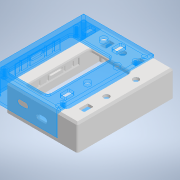
# Autodesk Inventor part: Frontpanel
Saved by Autodesk Inventor 2022 (Build 260153000, 153)
## iProperties
Created: 2020-11-05
Part Number: Frontpanel
Material: Generic
Document SubType Name: Modeling
Designer: simen
Density: 1 g/cm^3
Appearance: Default
Mass: 47.3769 g
Surface Area: 341.342 cm^2
Volume: 47.3769 cm^3
Author: simen
Autodesk Inventor part; units mm, degrees
ref_plane "YZ Plane" through (0, 0, 0) normal (1, 0, 0) x (0, 1, 0)
ref_plane "XZ Plane" through (0, 0, 0) normal (0, 1, 0) x (-1, 0, 0)
ref_plane "XY Plane" through (0, 0, 0) normal (0, 0, 1) x (1, 0, 0)
sketch "Sketch1" plane through (0, 0, 0) normal (0, 1, 0) x (-1, 0, 0)
  line L0 (-18.2777, 28.6513) -> (-98.2777, 28.6513)
  line L1 (-98.2777, 28.6513) -> (-98.2777, -79.3487)
  line L2 (-98.2777, -79.3487) -> (-18.2777, -79.3487)
  line L3 (-18.2777, -79.3487) -> (-18.2777, 28.6513)
  point P0 (0, 0)
  dimension "d0" = 80
  dimension "d42" = 108
  constraints: 8 end point, 2 parallel, 1 horizontal, 1 perpendicular
  measures "d0" distance of L2.end L1.end
  measures "d42" distance of L0.end L1.end
extrude "Extrusion1" add sketch "Sketch1" along normal blind 3
sketch "Sketch2" plane through (0, 3, 0) normal (0, 1, 0) x (1, 0, 0)
  line L0 (23.2777, -23.6513) -> (72.1777, -23.6513)
  line L1 (72.1777, -23.6513) -> (72.1777, 49.7887)
  line L2 (72.1777, 49.7887) -> (23.2777, 49.7887)
  line L3 (23.2777, 49.7887) -> (23.2777, -23.6513)
  line L4 (18.2777, 79.3487) -> (18.2777, -28.6513) projected
  line L5 (18.2777, -28.6513) -> (98.2777, -28.6513) projected
  line L6 (98.2777, 79.3487) -> (18.2777, 79.3487) projected
  point P0 (0, 0)
  dimension "d5" = 5
  dimension "d6" = 5
  dimension "d8" = 48.9
  dimension "d9" = 73.44
  constraints: 8 end point, 2 parallel, 1 horizontal, 1 perpendicular
  measures "d5" distance between parallel lines of L4 L3
  measures "d6" distance between parallel lines of L5 L0
  measures "d8" distance of L0.start L0.end
  measures "d9" distance between parallel lines of L2 L0
extrude "Extrusion2" [suppressed]
sketch "Sketch5" plane through (0, 0, 0) normal (0, -1, 0) x (1, 0, 0)
  line L0 (98.2777, 28.6513) -> (98.2777, -79.3487) projected
  line L1 (18.2777, 28.6513) -> (98.2777, 28.6513) projected
  line L2 (18.2777, -79.3487) -> (18.2777, 28.6513) projected
  line L3 (98.2777, -79.3487) -> (18.2777, -79.3487) projected
  line L4 (95.2777, 25.6513) -> (95.2777, -76.3487)
  line L5 (95.2777, -76.3487) -> (21.2777, -76.3487)
  line L6 (21.2777, -76.3487) -> (21.2777, 25.6513)
  line L7 (21.2777, 25.6513) -> (95.2777, 25.6513)
  point P0 (0, 0)
  dimension "d26" = 3
  constraints: 8 end point, 3 other
  measures "d26" distance between parallel lines of L1 L7
extrude "Extrusion7" add sketch "Sketch5" along normal blind 26
chamfer "Chamfer2" [suppressed]
fillet "Fillet2" radius 2 4 edges at (18.2777, -11.5, -79.3487) (98.2777, -11.5, -79.3487) (98.2777, -11.5, 28.6513) (18.2777, -11.5, 28.6513)
sketch "Sketch8" plane through (18.2777, -26, -77.3487) normal (-1, 0, 0) x (0, 0, 1)
  line L0 (57, 14.5) -> (47, 14.5) construction
  line L1 (57, 17) -> (47, 17)
  line L2 (47, 12) -> (57, 12)
  arc A0 (57, 12) -> (57, 17) centre (57, 14.5) ccw
  arc A1 (47, 17) -> (47, 12) centre (47, 14.5) ccw
  line L3 (0, 0) -> (0, 29) projected
  line L4 (104, 0) -> (0, 0) projected
  line L5 (104, 29) -> (104, 0) projected
  line L6 (104, 0) -> (0, 0) construction
  line L7 (48.7646, 0) -> (45.2354, 29) construction
  line L8 (0, 29) -> (104, 29) projected
  line L9 (0, 29) -> (104, 29) construction
  line L10 (104, 0) -> (0, 29) construction
  line L11 (0, 0) -> (0, 29) construction
  line L12 (0, 0) -> (104, 29) construction
  point P0 (52, 14.5)
  point P1 (52, 14.5)
  dimension "d51" = 10
  dimension "d52" = 5
  constraints: 14 end point, 4 point on circle, 4 tangent, 3 midpoint, 2 centre point, 1 coincident, 1 horizontal, 1 parallel, 1 point on line
  measures "d51" distance of L0.end L0.start
  measures "d52" diameter of A1
extrude "Extrusion9" cut sketch "Sketch8" against normal blind 10 contours A0 L2 A1 L1
sketch "Sketch9" plane through (0, 3, 0) normal (0, 1, 0) x (1, 0, 0)
  line L0 (35.2777, -20.6513) -> (75.2777, -20.6513)
  line L1 (78.2777, -17.6513) -> (78.2777, 48.3487)
  line L2 (75.2777, 51.3487) -> (35.2777, 51.3487)
  line L3 (32.2777, 48.3487) -> (32.2777, -17.6513)
  line L4 (18.2777, 69.3487) -> (18.2777, -25.6513) projected
  arc A0 (32.2777, -17.6513) -> (35.2777, -20.6513) centre (35.2777, -17.6513) ccw
  arc A1 (75.2777, -20.6513) -> (78.2777, -17.6513) centre (75.2777, -17.6513) ccw
  arc A2 (78.2777, 48.3487) -> (75.2777, 51.3487) centre (75.2777, 48.3487) ccw
  arc A3 (35.2777, 51.3487) -> (32.2777, 48.3487) centre (35.2777, 48.3487) ccw
  line L5 (98.2777, -26.6513) -> (98.2777, 77.3487) projected
  line L6 (20.2777, -28.6513) -> (96.2777, -28.6513) projected
  point P0 (0, 0)
  point P1 (78.2777, 51.3487)
  point P2 (78.2777, -20.6513)
  point P3 (32.2777, 51.3487)
  dimension "d56" = 46
  dimension "d57" = 72
  dimension "d59" = 14
  dimension "d60" = 3
  dimension "d116" = 20
  dimension "d144" = 8
  constraints: 8 end point, 8 point on circle, 8 tangent, 6 point on line, 4 centre point, 3 equal radius, 2 parallel, 1 horizontal, 1 perpendicular
  measures "d56" distance of point (32.278, 51.349) point (78.278, 51.349)
  measures "d57" distance of point (78.278, 51.349) point (78.278, -20.651)
  measures "d59" distance between parallel lines of L4 L3
  measures "d60" radius of A0
  measures "d116" distance between parallel lines of L5 L1
  measures "d144" distance between parallel lines of L6 L0
extrude "Extrusion10" cut sketch "Sketch9" against normal blind 10
chamfer "Chamfer4" distance 1 angle 45 8 edges at (33.1563, 3, 19.7726) (32.2777, 3, -15.3487) (33.1563, 3, -50.4701) (55.2777, 3, -51.3487) (77.399, 3, -50.4701) (78.2777, 3, -15.3487) (77.399, 3, 19.7726) (55.2777, 3, 20.6513)
chamfer "Chamfer5" distance 2 angle 45 8 edges at (98.2777, 3, -25.3487) (97.6919, 3, -78.763) (58.2777, 3, -79.3487) (18.8635, 3, -78.763) (18.2777, 3, -25.3487) (18.8635, 3, 28.0655) (58.2777, 3, 28.6513) (97.6919, 3, 28.0655)
fillet "Fillet3" radius 2 8 edges at (95.2777, -13, 25.6513) (95.2777, 0, -25.3487) (58.2777, 0, 25.6513) (95.2777, -13, -76.3487) (58.2777, 0, -76.3487) (21.2777, -13, -76.3487) (21.2777, 0, -25.3487) (21.2777, -13, 25.6513)
sketch "Sketch10" plane through (0, 3, 0) normal (0, 1, 0) x (1, 0, 0)
  arc A0 (31.2777, -17.6513) -> (35.2777, -21.6513) centre (35.2777, -17.6513) ccw projected
  line L0 (31.2777, 48.3487) -> (31.2777, -17.6513) projected
  arc A1 (35.2777, 52.3487) -> (31.2777, 48.3487) centre (35.2777, 48.3487) ccw projected
  line L1 (75.2777, 52.3487) -> (35.2777, 52.3487) projected
  arc A2 (79.2777, 48.3487) -> (75.2777, 52.3487) centre (75.2777, 48.3487) ccw projected
  line L2 (79.2777, -17.6513) -> (79.2777, 48.3487) projected
  arc A3 (75.2777, -21.6513) -> (79.2777, -17.6513) centre (75.2777, -17.6513) ccw projected
  line L3 (35.2777, -21.6513) -> (75.2777, -21.6513) projected
  line L4 (96.2777, -26.6513) -> (20.2777, -26.6513) projected
  line L5 (96.2777, 77.3487) -> (96.2777, -26.6513) projected
  line L6 (20.2777, 77.3487) -> (96.2777, 77.3487) projected
  line L7 (20.2777, -26.6513) -> (20.2777, 77.3487) projected
  arc A4 (75.2777, -21.6513) -> (79.2777, -17.6513) centre (75.2777, -17.6513) ccw projected
  line L8 (79.2777, -17.6513) -> (96.2777, -17.6513) construction
  line L9 (87.7777, -17.6513) -> (87.7777, -7.6513) construction
  circle A5 centre (87.7777, -7.6513) radius 2
  line L10 (87.7777, -7.6513) -> (87.7777, 17.3487) construction
  circle A6 centre (87.7777, 17.3487) radius 2
  point P0 (0, 0)
  dimension "d70" = 10
  dimension "d71" = 4
  dimension "d72" = 25
  dimension "d73" = 4
  constraints: 6 end point, 2 centre point, 2 coincident, 2 perpendicular, 1 collinear, 1 midpoint, 1 point on line
  measures "d70" distance of L9.start L9.end
  measures "d71" diameter of A5
  measures "d72" distance of L10.start L10.end
  measures "d73" diameter of A6
extrude "Extrusion11" [suppressed]
sketch "Sketch11" plane through (0, 0, 0) normal (0, -1, 0) x (1, 0, 0)
  circle A0 centre (92.2777, 22.6513) radius 2.5
  line L0 (95.2777, 23.6513) -> (95.2777, -74.3487) projected
  line L1 (23.2777, 25.6513) -> (93.2777, 25.6513) projected
  circle A1 centre (92.2777, -73.3487) radius 2.5
  circle A2 centre (24.2777, -73.3487) radius 2.5
  circle A3 centre (24.2777, 22.6513) radius 2.5
  line L2 (93.2777, -76.3487) -> (23.2777, -76.3487) projected
  line L3 (21.2777, -74.3487) -> (21.2777, 23.6513) projected
  point P0 (0, 0)
  dimension "d117" = 5
  dimension "d118" = 3
  dimension "d119" = 3
  dimension "d120" = 5
  dimension "d121" = 5
  dimension "d122" = 5
  dimension "d123" = 3
  dimension "d124" = 3
  dimension "d125" = 3
  dimension "d126" = 3
  dimension "d127" = 3
  dimension "d128" = 3
  constraints: 4 centre point
  measures "d117" diameter of A0
  measures "d118" distance from line of L0 A0.centre
  measures "d119" distance from line of L1 A0.centre
  measures "d120" diameter of A1
  measures "d121" diameter of A2
  measures "d122" diameter of A3
  measures "d123" distance from line of L0 A1.centre
  measures "d124" distance from line of L2 A1.centre
  measures "d125" distance from line of L2 A2.centre
  measures "d126" distance from line of L3 A2.centre
  measures "d127" distance from line of L1 A3.centre
  measures "d128" distance from line of L3 A3.centre
extrude "Extrusion13" add sketch "Sketch11" along normal blind 24
sketch "Sketch14" plane through (92.2777, -24, 22.6513) normal (0, -1, 0) x (1, 0, 0)
  circle A0 centre (0, 0) radius 2.5 projected
  circle A1 centre (0, -96) radius 2.5 projected
  circle A2 centre (-68, -96) radius 2.5 projected
  circle A3 centre (-68, 0) radius 2.5 projected
  circle A4 centre (0, -96) radius 1.5
  circle A5 centre (-68, -96) radius 1.5
  circle A6 centre (-68, 0) radius 1.5
  circle A7 centre (0, 0) radius 1.5
  point P0 (-92.2777, -22.6513)
  dimension "d138" = 1
  dimension "d139" = 1
  dimension "d140" = 1
  dimension "d141" = 1
  constraints: 4 centre point
  measures "d138" radial gap between concentric circles of A1 A4
  measures "d139" radial gap between concentric circles of A2 A5
  measures "d140" radial gap between concentric circles of A3 A6
  measures "d141" radial gap between concentric circles of A0 A7
extrude "Extrusion15" cut sketch "Sketch14" against normal blind 11 contours A4 | A5 | A6 | A7
sketch "Sketch15" plane through (0, 0, 0) normal (0, -1, 0) x (1, 0, 0)
  circle A0 centre (91.2777, 16.6513) radius 2.5
  circle A1 centre (25.2777, 16.6513) radius 2.5
  line L0 (23.2777, 25.6513) -> (93.2777, 25.6513) projected
  line L1 (95.2777, 23.6513) -> (95.2777, -74.3487) projected
  line L2 (21.2777, -74.3487) -> (21.2777, 23.6513) projected
  circle A2 centre (25.2777, -64.3487) radius 2.5
  circle A3 centre (91.2777, -64.3487) radius 2.5
  point P0 (0, 0)
  dimension "d145" = 5
  dimension "d146" = 5
  dimension "d147" = 9
  dimension "d148" = 9
  dimension "d149" = 4
  dimension "d150" = 4
  dimension "d151" = 5
  dimension "d152" = 5
  dimension "d153" = 4
  dimension "d154" = 4
  dimension "d155" = 90
  dimension "d156" = 90
  dimension "d166" = 66
  constraints: 4 centre point
  measures "d145" diameter of A0
  measures "d146" diameter of A1
  measures "d147" distance from line of L0 A0.centre
  measures "d148" distance from line of L0 A1.centre
  measures "d149" distance from line of L1 A0.centre
  measures "d150" distance from line of L2 A1.centre
  measures "d151" diameter of A2
  measures "d152" diameter of A3
  measures "d153" distance from line of L1 A3.centre
  measures "d154" distance from line of L2 A2.centre
  measures "d155" distance from line of L0 A2.centre
  measures "d156" distance from line of L0 A3.centre
  measures "d166" distance of A1.centre A0.centre
extrude "Extrusion16" add sketch "Sketch15" along normal blind 9.5
sketch "Sketch16" plane through (91.2777, -9.5, 16.6513) normal (0, -1, 0) x (1, 0, 0)
  circle A0 centre (0, 0) radius 2.5 projected
  circle A1 centre (0, -81) radius 2.5 projected
  circle A2 centre (-66, -81) radius 2.5 projected
  circle A3 centre (-66, 0) radius 2.5 projected
  point P0 (-91.2777, -16.6513)
hole "Hole2" at (91.2777, -9.5, 16.6513) at (91.2777, -9.5, -64.3487) at (25.2777, -9.5, -64.3487) at (25.2777, -9.5, 16.6513) direction (0, 1, 0) diameter 2.459 depth 8.8 tip angle 118 thread size "M3x0.5" class "6H" standard "ANSI Metric M Profile"
sketch "Sketch17" plane through (20.2777, -26, 28.6513) normal (0, 0, 1) x (1, 0, 0)
  line L0 (0, 27) -> (76, 27) projected
  line L1 (0, 0) -> (0, 27) projected
  line L2 (76, 0) -> (0, 0) projected
  line L3 (76, 27) -> (76, 0) projected
  line L4 (35, 13.6) -> (41, 13.6) construction
  line L5 (35, 11.6) -> (41, 11.6)
  line L6 (41, 15.6) -> (35, 15.6)
  arc A0 (35, 15.6) -> (35, 11.6) centre (35, 13.6) ccw
  arc A1 (41, 11.6) -> (41, 15.6) centre (41, 13.6) ccw
  point P0 (-20.2777, 26)
  point P1 (38, 13.6)
  dimension "d167" = 6
  dimension "d168" = 4
  dimension "d169" = 13.4
  dimension "d170" = 13.6
  dimension "d171" = 38
  dimension "d172" = 38
  constraints: 8 end point, 4 point on circle, 4 tangent, 2 centre point, 1 horizontal, 1 midpoint, 1 parallel
  measures "d167" distance of L4.start L4.end
  measures "d168" diameter of A1
  measures "d169" distance between parallel lines of L0 L4
  measures "d170" distance from line of L2 point (38, 13.6)
  measures "d171" distance from line of L1 point (38, 13.6)
  measures "d172" distance from line of L3 point (38, 13.6)
extrude "Extrusion17" cut sketch "Sketch17" against normal blind 4 contours A0 L6 A1 L5
chamfer "Chamfer6" distance 1 angle 45 4 edges at (58.2777, -10.4, 28.6513) (63.2777, -12.4, 28.6513) (58.2777, -14.4, 28.6513) (53.2777, -12.4, 28.6513)
sketch "Sketch18" plane through (0, 3, 0) normal (0, 1, 0) x (1, 0, 0)
  line L0 (79.2777, -17.6513) -> (79.2777, 48.3487) projected
  line L1 (96.2777, 77.3487) -> (96.2777, -26.6513) projected
  line L2 (79.2777, -17.6513) -> (96.2777, -17.6513)
  line L3 (78.2777, 48.3487) -> (79.2777, 48.3487) projected
  line L4 (79.2777, 48.3487) -> (95.2777, 48.3487)
  line L5 (95.2777, -23.6513) -> (95.2777, 74.3487) projected
  line L6 (79.2777, 15.3487) -> (95.2777, 15.3487)
  line L7 (87.2777, 15.3487) -> (79.2777, 15.3487)
  circle A0 centre (88.2777, 13.8487) radius 3.25
  circle A1 centre (88.2777, 46.8487) radius 3.25
  point P0 (0, 0)
  point P1 (96.2777, -26.6513)
  point P2 (97.2777, 77.3487)
  point P3 (97.2777, -26.6513)
  dimension "d178" = 6.5
  dimension "d179" = 6.5
  dimension "d191" = 8
  dimension "d192" = 8
  dimension "d193" = 31.5
  dimension "d194" = 1.5
  constraints: 8 end point, 2 centre point, 2 horizontal, 2 midpoint, 1 collinear, 1 parallel, 1 point on line, 2 other
  measures "d178" diameter of A0
  measures "d179" diameter of A1
  measures "d193" distance from line of L6 A1.centre
  measures "d194" distance from line of L6 A0.centre
extrude "Extrusion18" cut sketch "Sketch18" against normal blind 10 contours A0 L6 | L6 A0 | A1 L4 | L4 A1
sketch "Sketch19" plane through (0, 3, 0) normal (0, 1, 0) x (1, 0, 0)
  circle A0 centre (88.2777, 46.8487) radius 3.25 projected
  circle A1 centre (88.2777, 13.8487) radius 3.25 projected
  arc A2 (31.2777, -17.6513) -> (35.2777, -21.6513) centre (35.2777, -17.6513) ccw projected
  line L0 (31.2777, 48.3487) -> (31.2777, -17.6513) projected
  arc A3 (35.2777, 52.3487) -> (31.2777, 48.3487) centre (35.2777, 48.3487) ccw projected
  line L1 (75.2777, 52.3487) -> (35.2777, 52.3487) projected
  arc A4 (79.2777, 48.3487) -> (75.2777, 52.3487) centre (75.2777, 48.3487) ccw projected
  line L2 (79.2777, -17.6513) -> (79.2777, 48.3487) projected
  arc A5 (75.2777, -21.6513) -> (79.2777, -17.6513) centre (75.2777, -17.6513) ccw projected
  line L3 (35.2777, -21.6513) -> (75.2777, -21.6513) projected
  line L4 (96.2777, -26.6513) -> (20.2777, -26.6513) projected
  line L5 (96.2777, 77.3487) -> (96.2777, -26.6513) projected
  line L6 (20.2777, 77.3487) -> (96.2777, 77.3487) projected
  line L7 (20.2777, -26.6513) -> (20.2777, 77.3487) projected
  arc A6 (35.2777, 52.3487) -> (31.2777, 48.3487) centre (35.2777, 48.3487) ccw projected
  line L8 (31.2777, 48.3487) -> (31.2777, 77.3487)
  arc A7 (79.2777, 48.3487) -> (75.2777, 52.3487) centre (75.2777, 48.3487) ccw projected
  line L9 (79.2777, 48.3487) -> (79.2777, 77.3487)
  line L10 (20.2777, 77.3487) -> (96.2777, 77.3487) projected
  line L11 (35.2777, 52.3487) -> (35.2777, 77.3487)
  line L12 (75.2777, 52.3487) -> (75.2777, 77.3487)
  line L13 (75.2777, 64.8487) -> (35.2777, 64.8487)
  circle A8 centre (55.2777, 64.8487) radius 3.6
  line L14 (31.2777, 64.8487) -> (55.2777, 64.8487)
  circle A9 centre (38.2777, 64.8487) radius 3
  line L15 (55.2777, 64.8487) -> (79.2777, 64.8487)
  circle A10 centre (72.2777, 64.8487) radius 3
  line L16 (96.2777, 77.3487) -> (96.2777, -26.6513) projected
  line L17 (78.2777, -17.6513) -> (78.2777, 48.3487) projected
  line L18 (88.2777, 46.8487) -> (88.2777, 79.9428)
  line L19 (95.2777, 74.3487) -> (95.2777, -23.6513) projected
  line L20 (23.2777, 76.3487) -> (93.2777, 76.3487) projected
  line L21 (79.2777, -17.6513) -> (79.2777, 48.3487) projected
  line L22 (79.2777, 46.0388) -> (96.2777, 46.0388)
  line L23 (85.5277, -13.9013) -> (90.0277, -13.9013)
  line L24 (91.0277, -12.9013) -> (91.0277, -4.4013)
  line L25 (90.0277, -3.4013) -> (85.5277, -3.4013)
  line L26 (84.5277, -4.4013) -> (84.5277, -12.9013)
  line L27 (84.5277, -13.9013) -> (91.0277, -3.4013) construction
  line L28 (91.0277, -13.9013) -> (84.5277, -3.4013) construction
  arc A11 (84.5277, -12.9013) -> (85.5277, -13.9013) centre (85.5277, -12.9013) ccw
  arc A12 (90.0277, -13.9013) -> (91.0277, -12.9013) centre (90.0277, -12.9013) ccw
  arc A13 (91.0277, -4.4013) -> (90.0277, -3.4013) centre (90.0277, -4.4013) ccw
  arc A14 (85.5277, -3.4013) -> (84.5277, -4.4013) centre (85.5277, -4.4013) ccw
  line L29 (74.5277, 59.5987) -> (70.0277, 59.5987)
  line L30 (69.0277, 60.5987) -> (69.0277, 69.0987)
  line L31 (70.0277, 70.0987) -> (74.5277, 70.0987)
  line L32 (75.5277, 69.0987) -> (75.5277, 60.5987)
  line L33 (75.5277, 59.5987) -> (69.0277, 70.0987) construction
  line L34 (69.0277, 59.5987) -> (75.5277, 70.0987) construction
  line L35 (40.5277, 59.5987) -> (36.0277, 59.5987)
  line L36 (35.0277, 60.5987) -> (35.0277, 69.0987)
  line L37 (36.0277, 70.0987) -> (40.5277, 70.0987)
  line L38 (41.5277, 69.0987) -> (41.5277, 60.5987)
  line L39 (41.5277, 59.5987) -> (35.0277, 70.0987) construction
  line L40 (35.0277, 59.5987) -> (41.5277, 70.0987) construction
  arc A15 (35.0277, 60.5987) -> (36.0277, 59.5987) centre (36.0277, 60.5987) ccw
  arc A16 (36.0277, 70.0987) -> (35.0277, 69.0987) centre (36.0277, 69.0987) ccw
  arc A17 (41.5277, 69.0987) -> (40.5277, 70.0987) centre (40.5277, 69.0987) ccw
  arc A18 (40.5277, 59.5987) -> (41.5277, 60.5987) centre (40.5277, 60.5987) ccw
  arc A19 (69.0277, 60.5987) -> (70.0277, 59.5987) centre (70.0277, 60.5987) ccw
  arc A20 (70.0277, 70.0987) -> (69.0277, 69.0987) centre (70.0277, 69.0987) ccw
  arc A21 (75.5277, 69.0987) -> (74.5277, 70.0987) centre (74.5277, 69.0987) ccw
  arc A22 (74.5277, 59.5987) -> (75.5277, 60.5987) centre (74.5277, 60.5987) ccw
  line L41 (98.2777, -26.6513) -> (98.2777, 77.3487) projected
  point P0 (0, 0)
  point P1 (86.949, 59.6109)
  point P2 (88.2777, 58.5987)
  point P3 (35.2777, 64.8487)
  point P4 (41.2777, 64.8487)
  point P5 (75.2777, 64.8487)
  point P6 (69.2777, 64.8487)
  dimension "d182" = 7.2
  dimension "d183" = 6
  dimension "d184" = 6
  dimension "d189" = 17
  dimension "d190" = 17
  dimension "d200" = 10.5
  dimension "d201" = 1
  dimension "d202" = 6.5
  dimension "d203" = 10.5
  dimension "d204" = 6.5
  dimension "d205" = 10.5
  dimension "d206" = 1
  dimension "d207" = 6.5
  dimension "d208" = 17.25
  dimension "d209" = 7.25
  constraints: 54 end point, 35 point on line, 25 tangent, 24 point on circle, 15 centre point, 10 equal radius, 9 perpendicular, 7 midpoint, 7 parallel, 3 horizontal
  measures "d182" diameter of A8
  measures "d183" diameter of A9
  measures "d184" diameter of A10
  measures "d189" distance of A9.centre L14.end
  measures "d190" distance of L14.end A10.centre
  measures "d200" distance of L27.end L28.start
  measures "d201" radius of A11
  measures "d202" distance of L33.end L34.end
  measures "d203" distance of L34.start L33.end
  measures "d204" distance of L39.end L40.end
  measures "d205" distance of L40.start L39.end
  measures "d206" radius of A15
  measures "d207" distance between parallel lines of L24 L26
  measures "d208" distance from line of A1.centre L25
  measures "d209" distance between parallel lines of L41 L24
extrude "Extrusion19" cut sketch "Sketch19" against normal blind 10 contours L32 A22 L12 L15 | L15 L12 A21 L32 | L12 A10 L13 L30 A20 L31 A21 | A22 L29 A19 L30 L13 A10 L12 | A10 L13 | L13 A10 | A16 L37 A17 L38 L13 A9 L11 | L11 L14 L36 A16 | A15 L36 L14 L11 | L11 A9 L13 L38 A18 L35 A15 | A9 L13 | L13 A9 | A8 L13 | L13 A8 | A11 L26 A14 L25 A13 L24 A12 L23
sketch "Sketch20" plane through (21.2777, -26, 23.6513) normal (1, 0, 0) x (0, 0, -1)
  line L0 (0, 0) -> (0, 24) projected
  line L1 (98, 0) -> (0, 0) projected
  line L2 (98, 24) -> (98, 0) projected
  line L3 (0, 24) -> (98, 24) projected
  line L4 (54, 12) -> (44, 12) projected
  arc A0 (44, 17) -> (44, 12) centre (44, 14.5) ccw projected
  line L5 (44, 17) -> (54, 17) projected
  arc A1 (54, 12) -> (54, 17) centre (54, 14.5) ccw projected
  line L6 (74, 7.5) -> (24, 7.5)
  line L7 (24, 7.5) -> (24, 18.75)
  line L8 (24, 18.75) -> (74, 18.75)
  line L9 (74, 18.75) -> (74, 7.5)
  point P0 (23.6513, 26)
  dimension "d211" = 4.25
  dimension "d212" = 20
  dimension "d213" = 20
  dimension "d214" = 7
  constraints: 8 end point, 2 parallel, 1 horizontal, 1 perpendicular
  measures "d211" distance from line of L8 A1.centre
  measures "d212" distance from line of L9 A1.centre
  measures "d213" distance from line of L7 A0.centre
  measures "d214" distance from line of L6 A0.centre
extrude "Extrusion20" cut sketch "Sketch20" against normal blind 1 contours L6 L7 L8 L9
chamfer "Chamfer7" distance 1 angle 45 1 edges at (20.2777, -18.5, -25.3487)
sketch "Sketch22" plane through (21.2777, -7.25, -50.3487) normal (0, -1, 0) x (1, 0, 0)
  circle A0 centre (-1, 6.3) radius 1.05
  line L0 (0, 50) -> (0, 0) projected
  line L1 (0, 50) -> (-1, 50) projected
  line L2 (-1, 50) -> (-1, 0) projected
  line L3 (0, 0) -> (-1, 0) projected
  line L4 (-1, 50) -> (-1, 0) projected
  circle A1 centre (-1, 43.7) radius 1.05
  line L5 (0, 50) -> (0, 0) projected
  line L6 (0, 0) -> (0, 50) projected
  line L7 (0, -24) -> (0, 74) projected
  line L8 (0, 74) -> (0, -24) projected
  circle A2 centre (-1, 34.3) radius 1.05
  circle A3 centre (-1, 15.7) radius 1.05
  point P0 (-21.2777, 50.3487)
  point P1 (-1, 42.65)
  point P2 (-1, 44.75)
  point P3 (-1, 33.25)
  point P4 (-1, 35.35)
  point P5 (-1, 14.65)
  point P6 (-1, 16.75)
  point P7 (-1, 5.25)
  point P8 (-1, 7.35)
  dimension "d222" = 2.1
  dimension "d223" = 6.3
  dimension "d224" = 2.1
  dimension "d225" = 6.3
  dimension "d226" = 2.1
  dimension "d227" = 15.7
  dimension "d228" = 2.1
  dimension "d229" = 15.7
  constraints: 4 centre point, 4 point on line
  measures "d222" diameter of A0
  measures "d223" distance from line of L3 A0.centre
  measures "d224" diameter of A1
  measures "d225" distance from line of L1 A1.centre
  measures "d226" diameter of A2
  measures "d227" distance from line of L1 A2.centre
  measures "d228" diameter of A3
  measures "d229" distance from line of L3 A3.centre
extrude "Extrusion22" cut sketch "Sketch22" along normal up to surface contours L2 A0 | A3 L2 | A2 L2 | A1 L2 surface through (20.7777, -18, -37.8487) normal (0.7071068, 0.7071068, 0)
chamfer "Chamfer8" distance 0.2 angle 45 8 edges at (20.2777, -12.375, -45.0987) (20.2777, -12.375, -42.9987) (20.2777, -12.375, -35.6987) (20.2777, -12.375, -33.5987) (20.2777, -12.375, -17.0987) (20.2777, -12.375, -14.9987) (20.2777, -12.375, -7.6987) (20.2777, -12.375, -5.5987)
sketch "Sketch23" plane through (93.2777, -26, 25.6513) normal (0, 0, -1) x (-1, 0, 0)
  line L0 (32, 15.6) -> (38, 15.6) projected
  arc A0 (38, 11.6) -> (38, 15.6) centre (38, 13.6) ccw projected
  line L1 (38, 11.6) -> (32, 11.6) projected
  arc A1 (32, 15.6) -> (32, 11.6) centre (32, 13.6) ccw projected
  line L2 (0, 0) -> (0, 24) projected
  line L3 (70, 0) -> (0, 0) projected
  line L4 (70, 24) -> (70, 0) projected
  line L5 (0, 24) -> (70, 24) projected
  arc A2 (38, 11.6) -> (38, 15.6) centre (38, 13.6) ccw projected
  line L6 (40, 13.6) -> (40, 2)
  arc A3 (32, 15.6) -> (32, 11.6) centre (32, 13.6) ccw projected
  line L7 (30, 13.6) -> (30, 2)
  line L8 (30, 2) -> (40, 2)
  point P0 (93.2777, 26)
  dimension "d241" = 2
  constraints: 6 end point, 4 point on circle, 3 tangent, 2 vertical, 1 parallel
  measures "d241" distance between parallel lines of L3 L8
extrude "Extrusion23" cut sketch "Sketch23" against normal blind 0.75 contours A1 L1 A0 L6 L8 L7
chamfer "Chamfer9" distance 0.75 angle 45 1 edges at (58.2777, -24, 26.4013)
body "Solid1"
